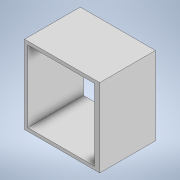
# Autodesk Inventor part: caja conexion
Saved by Autodesk Inventor 2020.3 (Build 243373000, 373)
## iProperties
Created: 2021-02-11
Part Number: caja conexion
Material: Generic
Document SubType Name: Modeling
Designer: Yu Jinyu
Density: 1 g/cm^3
Appearance: Default
Author: Yu Jinyu
Autodesk Inventor part; units mm, degrees
ref_plane "YZ Plane" through (0, 0, 0) normal (1, 0, 0) x (0, 1, 0)
ref_plane "XZ Plane" through (0, 0, 0) normal (0, 1, 0) x (-1, 0, 0)
ref_plane "XY Plane" through (0, 0, 0) normal (0, 0, 1) x (1, 0, 0)
sketch "Sketch1" plane through (0, 0, 0) normal (0, 0, 1) x (1, 0, 0)
  line L0 (-50.984, -54.6745) -> (50.984, -54.6745)
  line L1 (50.984, -54.6745) -> (50.984, 54.6745)
  line L2 (50.984, 54.6745) -> (-50.984, 54.6745)
  line L3 (-50.984, 54.6745) -> (-50.984, -54.6745)
  line L4 (-50.984, -54.6745) -> (50.984, 54.6745) construction
  line L5 (50.984, -54.6745) -> (-50.984, 54.6745) construction
  line L6 (-55.984, 59.6745) -> (55.984, 59.6745)
  line L7 (55.984, 59.6745) -> (55.984, -59.6745)
  line L8 (55.984, -59.6745) -> (-55.984, -59.6745)
  line L9 (-55.984, -59.6745) -> (-55.984, 59.6745)
  point P0 (0, 0)
  dimension "d0" = 101.968
  dimension "d1" = 109.349
  dimension "d2" = 5
  constraints: 20 end point, 4 parallel, 2 midpoint, 2 perpendicular, 1 horizontal, 3 other
  measures "d0" distance of L2.end L1.end
  measures "d1" distance of L1.end L0.end
  measures "d2" distance between parallel lines of L2 L6
extrude "Extrusion1" add sketch "Sketch1" along normal blind 50
sketch "Sketch5" plane through (50.984, -54.6745, 0) normal (-1, 0, 0) x (0, 0, 1)
  line L0 (0, -5) -> (50, -5) projected
  line L1 (0, 114.349) -> (50, 114.349) projected
  circle A0 centre (25, 54.6745) radius 9.525
  line L2 (50, 114.349) -> (50, -5) projected
  point P0 (0, 54.6745)
  dimension "d14" = 119.349
  dimension "d15" = 19.05
  dimension "d16" = 25
  dimension "d17" = 59.6745
  constraints: 1 centre point
  measures "d14" distance between parallel lines of L0 L1
  measures "d15" diameter of A0
  measures "d16" distance from line of A0.centre L2
  measures "d17" distance from line of L1 A0.centre
extrude "Extrusion5" cut sketch "Sketch5" against normal blind 2.778
sketch "Sketch6" plane through (55.984, -59.6745, 0) normal (1, 0, 0) x (0, 0, -1)
  line L0 (0, 0) -> (0, 119.349) projected
  line L1 (0, 119.349) -> (-50, 119.349) projected
  line L2 (-50, 0) -> (-50, 119.349) projected
  line L3 (0, 0) -> (-50, 0) projected
  point P0 (0, 59.6745)
extrude "Extrusion6" add sketch "Sketch6" along normal blind 2.778
sketch "Sketch7" plane through (53.762, 0, 25) normal (-1, 0, 0) x (0, 0, 1)
  circle A0 centre (0, 0) radius 9.525 projected
  circle A1 centre (0, 0) radius 7.495
  point P0 (-25, 0)
  dimension "d22" = 14.99
  constraints: 1 centre point, 1 coincident
  measures "d22" diameter of A1
extrude "Extrusion7" cut sketch "Sketch7" against normal blind 3 contours A1
sketch "Sketch8" plane through (0, 0, 0) normal (0, 0, -1) x (-1, 0, 0)
  line L0 (55.984, -59.6745) -> (-58.762, -59.6745) projected
  line L1 (55.984, 59.6745) -> (55.984, -59.6745) projected
  line L2 (55.984, 59.6745) -> (-58.762, 59.6745) projected
  line L3 (-58.762, -59.6745) -> (-58.762, 59.6745) projected
  line L4 (50.984, -54.6745) -> (50.984, 54.6745) projected
  line L5 (-50.984, -54.6745) -> (50.984, -54.6745) projected
  line L6 (-50.984, 54.6745) -> (-50.984, -54.6745) projected
  line L7 (50.984, 54.6745) -> (-50.984, 54.6745) projected
  point P0 (0, 0)
extrude "Extrusion8" add sketch "Sketch8" along normal blind 17.5
sketch "Sketch9" plane through (0, 0, 50) normal (0, 0, 1) x (1, 0, 0)
  line L0 (-55.984, -59.6745) -> (58.762, -59.6745) projected
  line L1 (58.762, 59.6745) -> (58.762, -59.6745) projected
  line L2 (-55.984, 59.6745) -> (58.762, 59.6745) projected
  line L3 (-55.984, 59.6745) -> (-55.984, -59.6745) projected
  line L4 (-50.984, -54.6745) -> (-50.984, 54.6745) projected
  line L5 (-50.984, 54.6745) -> (50.984, 54.6745) projected
  line L6 (50.984, 54.6745) -> (50.984, -54.6745) projected
  line L7 (50.984, -54.6745) -> (-50.984, -54.6745) projected
  point P0 (0, 0)
extrude "Extrusion9" add sketch "Sketch9" along normal blind 17.5
body "Solid1"
